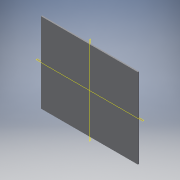
# Autodesk Inventor part: Convex Organ Bank Plate
Saved by Autodesk Inventor 2019 (Build 230136000, 136)
## iProperties
Created: 2021-02-18
Part Number: Convex Organ Bank Plate
Material: Generic
Document SubType Name: Modeling
Designer: Eric
Density: 1 g/cm^3
Appearance: Default
Author: Eric
Autodesk Inventor part; units mm, degrees
ref_plane "YZ Plane" through (0, 0, 0) normal (1, 0, 0) x (0, 1, 0)
ref_plane "XZ Plane" through (0, 0, 0) normal (0, 1, 0) x (-1, 0, 0)
ref_plane "XY Plane" through (0, 0, 0) normal (0, 0, 1) x (1, 0, 0)
sketch "Sketch1" plane through (0, 0, 0) normal (0, 0, 1) x (1, 0, 0)
  line L0 (0, 0) -> (400, 0)
  line L1 (400, 0) -> (400, -330)
  line L2 (400, -330) -> (0, -330)
  line L3 (0, -330) -> (0, 0)
  dimension "d0" = 400
  dimension "d1" = 330
  constraints: 8 end point, 2 horizontal, 2 vertical
  measures "d0" distance of L1.end L2.end
  measures "d1" distance of L0.end L1.end
extrude "Extrusion1" add sketch "Sketch1" along normal blind 5
ref_plane "Work Plane1" through (200, -330, 0) normal (1, 0, 0) x (0, 0, -1)
ref_plane "Work Plane2" through (0, -165, 0) normal (0, 1, 0) x (1, 0, 0)
body "Solid1"
